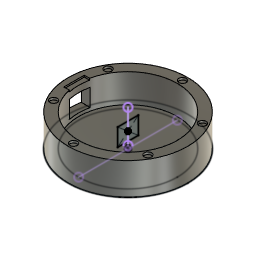
casev3 v10 (Autodesk Fusion 360 design; units mm, degrees)
Autodesk Fusion 360 part; units mm, degrees
sketch "Sketch1" plane through (0, 0, 0) normal (0, 0, 1) x (1, 0, 0) in component "Base"
  circle A0 centre (0, 0) radius 31
  circle A1 centre (0, 0) radius 37.5
  dimension "d8" = 62
  dimension "d9" = 75
  constraint coincident A0.centre A1.centre
  measures "d8" diameter of A0
  measures "d9" diameter of A1
extrude "Extrude2" add sketch "Sketch1" along normal blind 2 contours A0 makes body 1 in component "Base"
extrude "Extrude6" add sketch "Sketch1" along normal blind 20 bodies 1 in component "Base"
sketch "Sketch3" plane through (0, 0, 0) normal (1, 0, 0) x (0, 1, 0) in component "Base"
  line L0 (-6.5, 4) -> (6.5, 4)
  line L1 (6.5, 4) -> (6.5, 15)
  line L2 (6.5, 15) -> (-6.5, 15)
  line L3 (-6.5, 15) -> (-6.5, 4)
  line L4 (-6.5, 4) -> (6.5, 15) construction
  line L5 (6.5, 4) -> (-6.5, 15) construction
  line L6 (31, 0) -> (-31, 0)
  line L7 (0, 1.75) -> (0, 22.5)
  point P0 (0, 9.5)
  dimension "d18" = 13
  dimension "d19" = 11
  dimension "d20" = 4
  constraint horizontal L0
  constraint perpendicular L0 L1
  constraint parallel L0 L2
  constraint parallel L1 L3
  constraint coincident L4 P0
  constraint coincident L5 P0
  constraint symmetric L1 L3 L7
  measures "d18" distance of L0.start L0.end
  measures "d19" distance of L0.end L1.end
  measures "d20" distance of L0 L6
extrude "Extrude7" cut sketch "Sketch3" against normal blind 45 bodies 1 in component "Base"
sketch "Sketch1 (2)" plane through (0, 0, 20) normal (0, 0, 1) x (-1, 0, 0) in component "Tampa"
  circle A0 centre (0, 0) radius 31
  circle A1 centre (0, 0) radius 37.5
  circle A2 centre (0, 0) radius 37.5
  circle A3 centre (0, 0) radius 31
  circle A4 centre (0, 0) radius 22.8
  dimension "d103" = 45.6
  constraint concentric A3 A4
  measures "d103" diameter of A4
extrude "Extrude6'" add sketch "Sketch1 (2)" along normal blind 6 separate body contours A4 makes body 2 in component "Tampa"
extrude "Extrude1" add sketch "Sketch1 (2)" along normal blind 4 separate body contours A0 A3 | A1 A2 | A4 makes body 3 in component "Tampa"
sketch "Sketch2" plane through (0, 0, 26) normal (0, 0, 1) x (-1, 0, 0) in component "Tampa"
  circle A0 centre (0, 0) radius 31
  circle A1 centre (0, 0) radius 31
  circle A2 centre (0, 0) radius 10
  circle A3 centre (0, 0) radius 22.8
  dimension "d79" = 20
  constraint concentric A1 A2
  measures "d79" diameter of A2
fillet "Fillet3" radius 1 1 edges at (34.9623, 13.5606, 24) on bodies 3 in component "Tampa"
fillet "Fillet1" radius 1 4 edges at (-36.9324, -6.5, 9.5) (-37.5, 0, 4) (-36.9324, 6.5, 9.5) (-37.5, 0, 15) on bodies 1 in component "Base"
sketch "Sketch3 (2)" plane through (0, 0, 20) normal (0, 0, 1) x (-1, 0, 0) in component "Tampa"
  circle A0 centre (0, 0) radius 31
  line L0 (0, 0) -> (0, -43.3021) construction
  circle A1 centre (0, 0) radius 34.25 construction
  circle A2 centre (0, -34.25) radius 2.3
  circle A3 centre (29.6614, -17.125) radius 2.3
  circle A4 centre (29.6614, 17.125) radius 2.3
  circle A5 centre (0, 34.25) radius 2.3
  circle A6 centre (-29.6614, 17.125) radius 2.3
  circle A7 centre (-29.6614, -17.125) radius 2.3
  dimension "d90" = 68.5
  dimension "d91" = 4.6
  dimension "d93" = 360
  constraint coincident A0.centre L0.start
  constraint vertical L0
  constraint coincident L0 A2.centre
  constraint coincident A1 A2.centre
  measures "d90" diameter of A1
  measures "d91" diameter of A2
extrude "Extrude8" cut sketch "Sketch3 (2)" against normal blind 1.4 contours A2 | A3 | A4 | A5 | A6 | A7 bodies 1 in component "Base"
extrude "Extrude4" cut sketch "Sketch3 (2)" along normal blind 2.6 contours A2 | A3 | A4 | A5 | A6 | A7 bodies 3 in component "Tampa"
sketch "Sketch4" plane through (0, 0, 24) normal (0, 0, 1) x (-1, 0, 0) in component "Tampa"
  circle A0 centre (0, 0) radius 36.5
  circle A1 centre (0, 0) radius 36.5
  circle A2 centre (0, 0) radius 32.5 construction
  line L0 (34.7913, -6.2388) -> (30.2375, -6.2388)
  line L1 (30.2375, -6.2388) -> (30.2375, 6.6941)
  line L2 (30.2375, 6.6941) -> (34.7913, 6.6941)
  line L3 (34.7913, 6.6941) -> (34.7913, -6.2388)
  dimension "d98" = -4
  constraint horizontal L0
  constraint vertical L1
  constraint horizontal L2
  constraint vertical L3
fillet "Fillet4" radius 1 1 edges at (21.2571, 8.2448, 26) on bodies 2 in component "Tampa"
sketch "Sketch5" plane through (0, 0, 26) normal (0, 0, 1) x (-1, 0, 0) in component "Tampa"
  circle A0 centre (0, 0) radius 21.8
  circle A1 centre (0, 0) radius 10
extrude "Extrude7'" cut sketch "Sketch2" against normal blind 2 contours A2 bodies 2 in component "Tampa"
fillet "Fillet5" radius 1 1 edges at (9.3233, -3.6162, 26) on bodies 2 in component "Tampa"
sketch "Sketch6" plane through (0, 0, 24) normal (0, 0, 1) x (-1, 0, 0) in component "Tampa"
  circle A0 centre (0, 0) radius 36.5
  line L0 (33.7316, -6.2527) -> (26.6151, -6.2527)
  line L1 (26.6151, -6.2527) -> (26.6151, 6.5893)
  line L2 (26.6151, 6.5893) -> (33.7316, 6.5893)
  line L3 (33.7316, 6.5893) -> (33.7316, -6.2527)
  constraint horizontal L0
  constraint vertical L1
  constraint horizontal L2
  constraint vertical L3
extrude "Extrude10" cut sketch "Sketch6" against normal blind 5 contours L0 L1 L2 L3 bodies 1 in component "Base"
extrude "Extrude8'" cut sketch "Sketch6" against normal blind 5 contours L0 L1 L2 L3 bodies 3 in component "Tampa"
sketch "Sketch7" plane through (0, 0, 20) normal (0, 0, -1) x (1, 0, 0) in component "Tampa"
  circle A0 centre (0, 0) radius 22.8
  circle A1 centre (0, 0) radius 10
  circle A2 centre (0, 0) radius 12
  dimension "d116" = 2
extrude "Extrude9" cut sketch "Sketch7" against normal blind 2.5 contours A1 | A2 bodies 2 3 in component "Tampa"
sketch "Sketch8" plane through (0, 0, 24) normal (0, 0, 1) x (-1, 0, 0) in component "Tampa"
  line L0 (26.6151, -6.2527) -> (26.6151, 6.5893)
  line L1 (26.6151, 6.5893) -> (33.7316, 6.5893)
  line L2 (33.7316, 6.5893) -> (33.7316, -6.2527)
  line L3 (33.7316, -6.2527) -> (26.6151, -6.2527)
  circle A0 centre (0, 0) radius 36.5
  line L4 (-35.6956, 26.5917) -> (-12.4775, 45.1797)
ref_plane "WorkPlane1" through (24.0865, -35.8857, 24) normal (0.62497, -0.780649, 0) x (-0.780649, -0.62497, 0) in component "Tampa"
sketch "Sketch9" plane through (24.0865, -35.8857, 24) normal (0.62497, -0.780649, 0) x (-0.780649, -0.62497, 0) in component "Tampa"
  line L0 (-37.8744, 4) -> (30.6256, 4)
  line L1 (-41.1244, 4) -> (33.8756, 4)
  line L2 (-41.1244, 1) -> (33.8756, 1)
  line L3 (2.4461, 4) -> (-3.5539, 4)
  line L4 (-3.5539, 4) -> (-3.5539, 2)
  line L5 (-3.5539, 2) -> (2.4461, 2)
  line L6 (2.4461, 2) -> (2.4461, 4)
  dimension "d120" = 6
  dimension "d121" = 2
  constraint horizontal L3
  constraint vertical L4
  constraint horizontal L5
  constraint vertical L6
  constraint coincident L1 L3.start
  measures "d120" distance of L3.start L3.end
  measures "d121" distance of L3.start L5.end
extrude "Extrude10'" cut sketch "Sketch9" against normal blind 7 bodies 3 in component "Tampa"
fillet "Fillet6" radius 1 3 edges at (20.9525, -31.1006, 22) (23.3813, -29.3183, 21) (18.3884, -32.6821, 21) on bodies 3 in component "Tampa"
extrude "Extrude9'" [suppressed] in component "Base"
component "Base" placed x (1, 0, 0) y (0, 1, 0) z (0, 0, 1) at (0, 0, 0)
component "Tampa" placed x (1, 0, 0) y (0, 1, 0) z (0, 0, 1) at (0, 0, 0)
equation "altura_interna = 20 mm"
equation "paredes_externas = 13 mm"
equation "led_interno = 48 mm"
equation "led_externo = 75 mm"
equation "folga = 0.6 mm"
equation "usb_largura = 13 mm"
equation "usb_altura = 11 mm"
equation "d8 = led_externo - paredes_externas"
equation "d9 = led_externo"
equation "paredes = 4 mm"
equation "d13 = paredes / 2"
equation "d18 = usb_largura"
equation "d19 = usb_altura"
equation "d20 = paredes"
equation "ima_largura = 4 mm"
equation "ima_altura = 2 mm"
equation "d71 = altura_interna"
equation "d90 = led_externo - 6.5 mm"
equation "d91 = ima_largura + folga"
equation "d94 = ima_altura + folga"
equation "d96 = -ima_altura + folga"
equation "d103 = led_interno - folga * 4"
named bodies: "Lateral"
